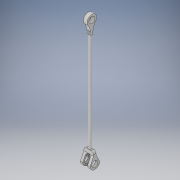
# Autodesk Inventor part: Connector_Rd
Saved by Autodesk Inventor 2019 (Build 230136000, 136)
## iProperties
Created: 2019-11-16
Part Number: Connector_Rd
Material: Generic
Document SubType Name: Modeling
Designer: Jorian Brusind
Density: 1 g/cm^3
Appearance: Default
Author: Jorian Brusind
Autodesk Inventor part; units mm, degrees
ref_plane "XY Plane" through (0, 0, 0) normal (0, 0, 1) x (1, 0, 0)
sketch "Sketch1" plane through (0, 0, 0) normal (0, 1, 0) x (-1, 0, 0)
  circle A0 centre (0, 0) radius 0.5
  dimension "d0" = 1
  constraints: 1 centre point, 1 coincident
  measures "d0" diameter of A0
extrude "Extrusion1" add sketch "Sketch1" along normal blind 45
sketch "Sketch2" plane through (0, 0, 0) normal (1, 0, 0) x (0, 1, 0)
  line L0 (45, -0.5) -> (45, 0.5) projected
  line L1 (45, 0) -> (48, 0)
  circle A0 centre (48, 0) radius 1.25
  circle A1 centre (48, 0) radius 2
  line L2 (0, 0.5) -> (45, 0.5) projected
  spline S0 degree 2 poles (48, 2) (44.0604, 0.0789) (42.6332, 0.5) knots 0 0 0 1 1 1
  line L3 (0, -0.5) -> (45, -0.5) projected
  spline S1 degree 2 poles (48.029, -1.9998) (44.0596, -0.0803) (42.6332, -0.5) knots 0 0 0 1 1 1
  line L4 (42.6332, 0.5) -> (42.6332, -0.5)
  point P0 (0, 0)
  point P1 (43.9843, 0.5)
  point P2 (43.9843, -0.5)
  dimension "d3" = 3
  dimension "d4" = 2.5
  dimension "d5" = 4
  constraints: 4 end point, 4 point on line, 2 centre point, 2 coincident, 2 point on circle, 1 horizontal, 1 midpoint, 1 vertical, 6 other
  measures "d3" distance of L1.start L1.end
  measures "d4" diameter of A0
  measures "d5" diameter of A1
extrude "Extrusion2" add sketch "Sketch2" along normal mid plane 1.5 contours L3 S1 L4 S0 L2 L0 | L0 L1 A1 S1 L3 | L0 L2 S0 A1 L1 | A1 S0 S1 | S1 A1 | A1 S0
ref_plane "Work Plane1" through (0, 29.4275, 0) normal (0, 1, 0) x (-1, 0, 0)
ref_plane "Work Plane2" through (1, 0, 0) normal (1, 0, 0) x (0, 1, 0)
sketch "Sketch3" plane through (1, 0, 0) normal (1, 0, 0) x (0, 1, 0)
  line L0 (0, 0) -> (-3, 0)
  circle A0 centre (-3, 0) radius 2
  line L1 (0, 0.5) -> (0, -0.5) projected
  spline S0 degree 2 poles (-3, 2) (-0.0143, 0.4702) (1.0884, 0) knots 0 0 0 1 1 1
  spline S1 degree 2 poles (-3, -2) (-0.0143, -0.4702) (1.0884, 0) knots 0 0 0 1 1 1
  circle A1 centre (-3, 0) radius 1.25
  dimension "d10" = 3
  dimension "d11" = 4
  dimension "d12" = 2.5
  constraints: 2 centre point, 2 coincident, 2 end point, 2 point on circle, 1 horizontal, 6 other
  measures "d10" distance of L0.start L0.end
  measures "d11" diameter of A0
  measures "d12" diameter of A1
extrude "Extrusion3" add sketch "Sketch3" along normal blind 1 contours L1 S1 A0 L0 | L0 A0 S0 L1 | A0 S1 S0
ref_plane "Work Plane3" through (0, 0, 0) normal (1, 0, 0) x (0, 1, 0)
mirror "Mirror2" about plane through (0, 0, 0) normal (1, 0, 0) of "Extrusion3"
sketch "Sketch4" plane through (2, 0, 0) normal (1, 0, 0) x (0, 0, -1)
  line L0 (0, 0) -> (0.5, 0) projected
  line L1 (-0.5, 0) -> (-0.5, 42.6332) projected
  line L2 (0.5, 0) -> (-0.5, 0)
  line L3 (-0.5, 0) -> (-0.5, 1.5)
  line L4 (-0.5, 1.5) -> (0.5, 1.5)
  line L5 (0.5, 1.5) -> (0.5, 0)
  dimension "d16" = 1.5
  constraints: 8 end point, 2 parallel, 1 horizontal, 1 perpendicular, 1 point on line
  measures "d16" distance of L2.end L3.end
extrude "Extrusion4" add sketch "Sketch4" against normal blind 4
fillet "Fillet1" radius 1 2 edges at (-1, 0, 0) (1, 0, 0)
fillet "Fillet3" radius 1 2 edges at (-2, 1.5, 0) (2, 1.5, 0)
body "Solid1"
